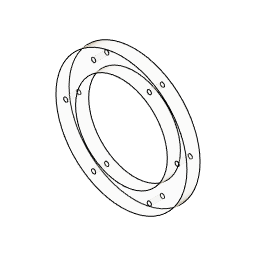
cone_fastener (Autodesk Fusion 360 design; units mm, degrees)
Autodesk Fusion 360 part; units mm, degrees
sketch "Esquisse1" plane through (0, 0, 0) normal (0, 1, 0) x (1, 0, 0)
  circle A0 centre (0, 0) radius 35
  circle A1 centre (0, 0) radius 50
  line L0 (42.5, 0) -> (21.25, 36.8061) construction
  line L1 (21.25, 36.8061) -> (-21.25, 36.8061) construction
  line L2 (-21.25, 36.8061) -> (-42.5, 0) construction
  line L3 (-42.5, 0) -> (-21.25, -36.8061) construction
  line L4 (-21.25, -36.8061) -> (21.25, -36.8061) construction
  line L5 (21.25, -36.8061) -> (42.5, 0) construction
  circle A2 centre (0, 0) radius 42.5 construction
  line L6 (50, 0) -> (-50, 0)
  line L7 (0, -50) -> (0, 50)
  circle A3 centre (21.25, -36.8061) radius 1.6
  circle A4 centre (-21.25, -36.8061) radius 1.6
  circle A5 centre (-42.5, 0) radius 1.6
  circle A6 centre (-21.25, 36.8061) radius 1.6
  circle A7 centre (21.25, 36.8061) radius 1.6
  circle A8 centre (42.5, 0) radius 1.6
  dimension "d1" = 70
  dimension "d2" = 15
  dimension "d5" = 7.5
  dimension "d6" = 3.2
  constraint coincident A0.centre A1.centre
  constraint coincident L4.end A2
  constraint coincident A1 L6.start
  constraint coincident A1 L6.end
  constraint horizontal L6
  constraint coincident A1 L7.start
  constraint coincident A1 L7.end
  constraint perpendicular L6 L7
  constraint coincident L0.start L6
  constraint coincident L4.end L5.start
  constraint coincident L3.end L4.start
  constraint coincident A0.centre L6
  constraint coincident L2.end L3.start
  constraint coincident L1.end L2.start
  constraint coincident L0.end L1.start
  constraint coincident L0.start L5.end
  constraint equal A3 A4
  constraint equal A3 A8
  constraint equal A7 A8
  constraint equal A4 A5
  constraint equal A6 A7
  measures "d1" diameter of A0
  measures "d2" distance of A0 A1
  measures "d5" distance of A0 A2
  measures "d6" diameter of A4
extrude "Extrusion1" add sketch "Esquisse1" along normal blind 10 contours A0 A1 L6 L7 A8 | A0 A1 L6 L7 A8 | A0 A1 L6 L7 A5 | A0 A1 L6 L7 A5
